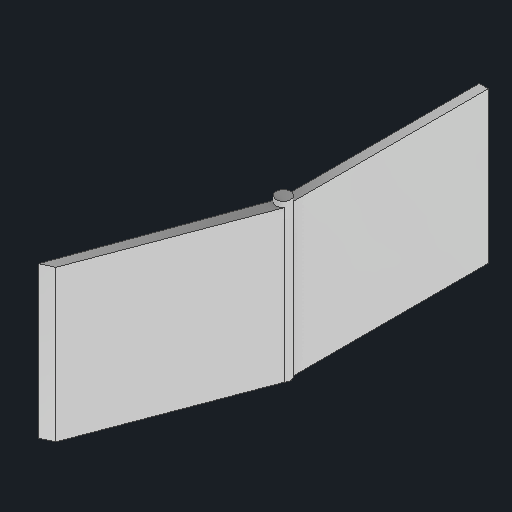
# Autodesk Inventor part: McCrea_finger_Walle
Saved by Autodesk Inventor 2022 (Build 260153000, 153)
## iProperties
Created: 2022-01-26
Part Number: McCrea_finger_Walle
Material: Generic
Document SubType Name: Modeling
Designer: Lukas
Density: 1 g/cm^3
Appearance: Chrome - Polished
Author: Lukas
Autodesk Inventor part; units mm, degrees
ref_plane "YZ Plane" through (0, 0, 0) normal (1, 0, 0) x (0, 1, 0)
ref_plane "XZ Plane" through (0, 0, 0) normal (0, 1, 0) x (-1, 0, 0)
ref_plane "XY Plane" through (0, 0, 0) normal (0, 0, 1) x (1, 0, 0)
sketch "Sketch1" plane through (0, 0, 0) normal (0, 1, 0) x (-1, 0, 0)
  line L0 (0, 0) -> (-5, 0)
  line L1 (-5, 0) -> (-5, 3.5)
  line L2 (-0.5, 3.5) -> (0, 3.5)
  line L3 (0, 3.5) -> (0, 0)
  line L4 (-5, 0) -> (-4.5, 0)
  line L5 (-4.5, 7.5) -> (-4.5, 11)
  line L6 (-4.5, 11) -> (-5, 11)
  line L7 (-5, 11) -> (-5, 0)
  arc A0 (-4.5, 7.5) -> (-0.5, 3.5) centre (-0.5, 7.5) ccw
  dimension "d0" = 5
  dimension "d1" = 3.5
  dimension "d2" = 0.5
  dimension "d3" = 11
  dimension "d4" = 4
  constraints: 16 end point, 4 parallel, 2 horizontal, 2 perpendicular, 2 point on circle, 2 point on line, 2 tangent, 1 centre point
  measures "d0" distance of L1.end L2.end
  measures "d1" distance of L0.end L1.end
  measures "d2" distance of L6.end L5.end
  measures "d3" distance of L5.end L4.end
  measures "d4" radius of A0
extrude "Extrusion1" add sketch "Sketch1" along normal blind 3.5
sketch "Sketch2" plane through (0, 3.5, 0) normal (0, 1, 0) x (1, 0, 0)
  line L0 (0, -3.5) -> (0.5, -3.5) projected
  line L1 (5, -11) -> (5, 0) projected
  line L2 (0, -3.5) -> (5, -3.5)
  line L3 (5, -3.5) -> (5, 0)
  line L4 (5, 0) -> (0, 0)
  line L5 (0, 0) -> (0, -3.5)
  circle A0 centre (1.551, -1.75) radius 0.75
  dimension "d7" = 1.5
  constraints: 8 end point, 2 parallel, 1 centre point, 1 horizontal, 1 perpendicular
  measures "d7" diameter of A0
extrude "Extrusion2" cut sketch "Sketch2" against normal blind 3.5 contours A0
sketch "Sketch3" plane through (0, 0, 0) normal (0, -1, 0) x (1, 0, 0)
  line L0 (5, 11) -> (5, 0) projected
  arc A0 (0.5, 3.5) -> (4.5, 7.5) centre (0.5, 7.5) ccw projected
  line L1 (5, 11) -> (4.5, 11)
  line L2 (4.5, 11) -> (4.5, 7.5)
  line L3 (4.5, 7.5) -> (5, 7.5)
  line L4 (5, 7.5) -> (5, 11)
  line L5 (5, 0) -> (0, 0) projected
  line L6 (5, 7.5) -> (4.5, 7.5)
  line L7 (4.5, 7.5) -> (4.5, 0)
  line L8 (4.5, 0) -> (5, 0)
  line L9 (5, 0) -> (5, 7.5)
  constraints: 16 end point, 4 parallel, 2 horizontal, 2 perpendicular, 2 point on line
extrude "Extrusion3" add sketch "Sketch3" along normal blind 4.8
sketch "Sketch4" plane through (0, 3.5, 0) normal (0, 1, 0) x (1, 0, 0)
  line L0 (5, -11) -> (4.5, -11) projected
  circle A0 centre (4.75, -11) radius 0.4
  point P0 (0, 0)
  dimension "d12" = 0.8
  constraints: 1 centre point, 1 midpoint
  measures "d12" diameter of A0
extrude "Extrusion4" add sketch "Sketch4" along normal blind 0.3 and the other way blind 8.3
sketch "Sketch5" plane through (0, -4.8, 0) normal (0, -1, 0) x (1, 0, 0)
  circle A0 centre (4.75, 11) radius 0.4 projected
  line L0 (4.6264, 10.6196) -> (0.9709, 20.663)
  line L1 (4.6264, 10.6196) -> (15.3144, 10.6196) construction
  line L2 (0.9709, 20.663) -> (1.4407, 20.834)
  line L3 (1.4407, 20.834) -> (5.0551, 11.2587)
  point P0 (0, 0)
  point P1 (4.4108, 11.212)
  dimension "d17" = 10.688
  dimension "d18" = 110
  dimension "d19" = 0.5
  constraints: 8 end point, 2 point on circle, 1 equal length, 1 horizontal
  measures "d17" distance of L0.start L0.end
  measures "d18" angle of L1 L0
  measures "d19" distance of L0.end L2.end
extrude "Extrusion5" add sketch "Sketch5" against normal blind 8.3 contours A0 L0 L2 L3
chamfer "Chamfer1" distance 0.5 angle 45 1 edges at (1.4407, -0.65, 20.834)
extrude "Extrusion6" add sketch "Sketch1" against normal blind 4.8
extrude "Extrusion7" cut sketch "Sketch2" against normal blind 10 contours A0
sketch "Sketch8" plane through (0, 3.5, 0) normal (0, 1, 0) x (1, 0, 0)
  arc A0 (4.5, -7.5) -> (0.5, -3.5) centre (0.5, -7.5) ccw projected
  line L0 (4.5, -7.5) -> (4.5, 0)
  line L1 (0, 0) -> (5, 0) projected
  line L2 (4.5, 0) -> (0, 0)
  line L3 (0, -3.5) -> (0, 0) projected
  line L4 (0, 0) -> (0, -3.5)
  line L5 (4.5, -10.6878) -> (4.5, -7.5) projected
  line L6 (0.5, -3.5) -> (0, -3.5) projected
  arc A1 (4.5, -7.5) -> (0, -3.5) centre (0.0283, -7.9995) ccw
  constraints: 6 end point, 2 collinear, 2 point on circle, 1 centre point, 1 vertical
extrude "Extrusion8" cut sketch "Sketch8" against normal blind 3.5
sketch "Sketch10" plane through (0, 0, 0) normal (0, 1, 0) x (1, 0, 0)
  arc A0 (4.5, -7.5) -> (0.5, -3.5) centre (0.5, -7.5) ccw projected
  line L0 (4.5, -7.5) -> (4.5, 0)
  line L1 (0, 0) -> (4.5, 0) projected
  line L2 (4.5, 0) -> (0, 0)
  line L3 (0, -3.5) -> (0, 0) projected
  line L4 (0, 0) -> (0, -3.5)
  arc A1 (0.0565, -3.5) -> (0, -3.5) centre (0.0283, -7.9995) ccw projected
  arc A2 (4.5, -7.5) -> (0, -3.5) centre (0.4527, -7.522) ccw
  point P0 (3.0783, -4.4418)
  constraints: 6 end point, 2 point on circle, 1 centre point, 1 collinear, 1 perpendicular, 1 tangent, 1 vertical
extrude "Extrusion9" cut sketch "Sketch10" against normal blind 1.3 contours A0 A2 L3 L1 L0
sketch "Sketch11" plane through (0, -1.3, 0) normal (0, 1, 0) x (1, 0, 0)
  line L0 (4.5, -7.5) -> (-4.9398, -7.5)
  line L1 (-4.9398, -7.5) -> (-4.9398, 2.7302)
  line L2 (-4.9398, 2.7302) -> (4.5, 2.7302)
  line L3 (4.5, 2.7302) -> (4.5, -7.5)
  point P0 (0, 0)
  constraints: 8 end point, 2 parallel, 1 horizontal, 1 perpendicular
extrude "Extrusion10" cut sketch "Sketch11" along normal blind 10
body "Solid1"
